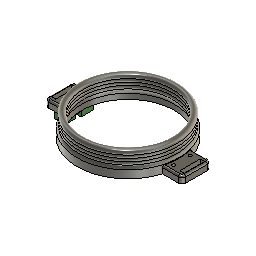
Lunette (Autodesk Fusion 360 design; units mm, degrees)
Autodesk Fusion 360 part; units mm, degrees
sketch "Sketch1" plane through (0, 0, 0) normal (0, 0, 1) x (1, 0, 0)
  circle A0 centre (0, 0) radius 64.5
  circle A1 centre (0, 0) radius 70.5
  line L0 (95, -20) -> (-95, -20)
  line L1 (-95, -20) -> (-95, 20)
  line L2 (-95, 20) -> (95, 20)
  line L3 (95, 20) -> (95, -20)
  line L4 (95, -20) -> (-95, 20) construction
  line L5 (-95, -20) -> (95, 20) construction
  line L6 (-67, 20) -> (-67, -20)
  line L7 (67, 20) -> (67, -20)
  line L8 (-83, 20) -> (-83, -20)
  line L9 (83, 20) -> (83, -20)
  line L10 (-83, 20) -> (-95, -20) construction
  line L11 (83, 20) -> (95, -20) construction
  line L12 (-86, -14) -> (-92, -14)
  line L13 (-92, -14) -> (-92, 14)
  line L14 (-92, 14) -> (-86, 14)
  line L15 (-86, 14) -> (-86, -14)
  line L16 (-86, -14) -> (-92, 14) construction
  line L17 (-92, -14) -> (-86, 14) construction
  line L18 (0, 20) -> (0, -20) construction
  line L19 (92, -14) -> (92, 14)
  line L20 (92, 14) -> (86, 14)
  line L21 (86, 14) -> (86, -14)
  line L22 (86, -14) -> (92, -14)
  line L23 (-89, 0) -> (0, 0) construction
  circle A2 centre (-75, -11.5) radius 2.1
  line L24 (-67, 20) -> (-83, -20) construction
  line L25 (-75, 20) -> (-75, -20) construction
  circle A3 centre (-75, 11.5) radius 2.1
  line L26 (75, 20) -> (75, -20) construction
  circle A4 centre (75, 11.5) radius 2.1
  circle A5 centre (75, -11.5) radius 2.1
  point P0 (-89, 0)
  dimension "d1" = 129
  dimension "d2" = 6
  dimension "d3" = 16
  dimension "d4" = 16
  dimension "d5" = 12
  dimension "d6" = 12
  dimension "d7" = 3
  dimension "d8" = 6
  dimension "d9" = 40
  dimension "d15" = 4.2
  dimension "d31" = 8.5
  dimension "d32" = 4.2
  dimension "d33" = 8.5
  dimension "d55" = 75
  dimension "d56" = 8
  constraint coincident A0.centre A1.centre
  constraint horizontal L0
  constraint perpendicular L0 L1
  constraint parallel L0 L2
  constraint parallel L1 L3
  constraint coincident L4 A0.centre
  constraint coincident L5 A0.centre
  constraint coincident L2 L6.start
  constraint coincident L0 L6.end
  constraint perpendicular L0 L6
  constraint coincident L2 L7.start
  constraint coincident L0 L7.end
  constraint perpendicular L0 L7
  constraint coincident L2 L8.start
  constraint coincident L0 L8.end
  constraint perpendicular L0 L8
  constraint coincident L2 L9.start
  constraint coincident L0 L9.end
  constraint perpendicular L0 L9
  constraint horizontal L12
  constraint perpendicular L12 L13
  constraint parallel L12 L14
  constraint parallel L13 L15
  constraint coincident L16 P0
  constraint coincident L17 P0
  constraint midpoint L10 P0
  constraint midpoint L2 L18.start
  constraint midpoint L0 L18.end
  constraint symmetric L12.start L18 L21.end
  constraint symmetric L12.end L18 L19.start
  constraint symmetric L13.end L18 L19.end
  constraint symmetric L14.end L18 L20.end
  constraint coincident P0 L23.start
  constraint coincident L2 L25.start
  constraint coincident L0 L25.end
  constraint perpendicular L0 L25
  constraint midpoint L24 L25
  constraint coincident A2.centre L25
  constraint coincident L25 A3.centre
  constraint symmetric L18 A2 A5
  constraint symmetric L18 L25.start L26.start
  constraint symmetric L18 L25.end L26.end
  constraint symmetric L18 A3 A4
  measures "d1" diameter of A0
  measures "d3" distance of L6.start L8.start
  measures "d4" distance of L7.start L9.start
  measures "d5" distance of L1 L8
  measures "d6" distance of L2.end L9.start
  measures "d7" horizontal distance of L1.end L13.end
  measures "d8" vertical distance of L1.end L13.end
  measures "d9" distance of L0.start L2.end
  measures "d15" diameter of A2
  measures "d31" distance of A2.centre L25.end
  measures "d32" diameter of A3
  measures "d33" distance of L25.start A3.centre
  measures "d55" distance of L18.start L25.start
  measures "d56" distance of L7.start L26.start
extrude "Extrude4" add sketch "Sketch1" along normal blind 15 contours A0 L0 L2 L7 | A0 A1 L2 | A0 A1 L0 | A0 L0 L2 L6 | A1 L0 L2 L7 | A1 L0 L2 L6 makes body 1
extrude "Extrude1" add sketch "Sketch1" along normal blind 10 contours A0 L0 L2 L7 | A0 A1 L2 | A0 A1 L0 | A0 L0 L2 L6 | A1 L0 L2 L7 | A1 L0 L2 L6 | A1 L0 L2 L9 | A1 L0 L2 L8 | L0 L2 L3 L9 | L0 L1 L2 L8 bodies 1
fillet "Fillet1" radius 5 4 edges at (95, -20, 5) (95, 20, 5) (-95, -20, 5) (-95, 20, 5) on bodies 1
fillet "Fillet2" radius 2.5 10 edges at (-78.8018, 20, 10) (-93.5355, 18.5355, 10) (-95, 0, 10) (-93.5355, -18.5355, 10) (-78.8018, -20, 10) (78.8018, -20, 10) (93.5355, -18.5355, 10) (95, 0, 10) (93.5355, 18.5355, 10) (78.8018, 20, 10) on bodies 1
sketch "Sketch2" plane through (0, 0, 10) normal (0, 0, 1) x (-1, 0, 0)
  line L0 (90, 17.5) -> (68.2935, 17.5)
  arc A0 (68.2935, -17.5) -> (68.2935, 17.5) centre (0, 0) ccw
  line L1 (68.2935, -17.5) -> (90, -17.5)
  arc A1 (90, -17.5) -> (92.5, -15) centre (90, -15) ccw
  line L2 (92.5, -15) -> (92.5, 15)
  arc A2 (92.5, 15) -> (90, 17.5) centre (90, 15) ccw
  circle A3 centre (75, -11.5) radius 2.1
  circle A4 centre (75, 11.5) radius 2.1
  line L3 (92, -14) -> (86, -14)
  line L4 (86, -14) -> (86, 14)
  line L5 (86, 14) -> (92, 14)
  line L6 (92, 14) -> (92, -14)
  circle A5 centre (75, 11.5) radius 3.75
  circle A6 centre (75, -11.5) radius 3.75
  line L7 (-90, -17.5) -> (-68.2935, -17.5)
  arc A7 (-68.2935, 17.5) -> (-68.2935, -17.5) centre (0, 0) ccw
  line L8 (-68.2935, 17.5) -> (-90, 17.5)
  arc A8 (-90, 17.5) -> (-92.5, 15) centre (-90, 15) ccw
  line L9 (-92.5, 15) -> (-92.5, -15)
  arc A9 (-92.5, -15) -> (-90, -17.5) centre (-90, -15) ccw
  circle A10 centre (-75, -11.5) radius 2.1
  line L10 (-92, 14) -> (-86, 14)
  line L11 (-86, 14) -> (-86, -14)
  line L12 (-86, -14) -> (-92, -14)
  line L13 (-92, -14) -> (-92, 14)
  circle A11 centre (-75, 11.5) radius 2.1
  circle A12 centre (-75, -11.5) radius 3.75
  circle A13 centre (-75, 11.5) radius 3.75
  dimension "d36" = 7.5
  dimension "d44" = 7.5
  dimension "d45" = 7.5
  dimension "d46" = 7.5
  constraint concentric A4 A5
  constraint concentric A3 A6
  constraint concentric A10 A12
  constraint concentric A11 A13
  measures "d36" diameter of A5
  measures "d44" diameter of A6
  measures "d45" diameter of A12
  measures "d46" diameter of A13
ref_plane "WorkPlane1" through (0, 0, 17) normal (0, 0, 1) x (1, 0, 0)
torus "TorusPrimitive3" add centre line diameter 130 section diameter 8 placed x (1, 0, 0) y (0, 1, 0) z (0, 0, 1) at (0, 0, 17) bodies 1
fillet "Fillet3" radius 5.5 1 edges at (-65.7291, -25.4939, 15) on bodies 1
ref_plane "WorkPlane2" through (0, 0, 21) normal (0, 0, 1) x (1, 0, 0)
torus "TorusPrimitive4" add centre line diameter 130 section diameter 8 placed x (1, 0, 0) y (0, 1, 0) z (0, 0, 1) at (0, 0, 21) bodies 1
ref_plane "WorkPlane3" through (0, 0, 25) normal (0, 0, 1) x (1, 0, 0)
torus "TorusPrimitive5" add centre line diameter 130 section diameter 8 placed x (1, 0, 0) y (0, 1, 0) z (0, 0, 1) at (0, 0, 25) bodies 1
fillet "Fillet4" radius 11 1 edges at (-60.1351, -23.3242, 13.0314) on bodies 1
ref_plane "WorkPlane4" through (0, 0, 29) normal (0, 0, 1) x (1, 0, 0)
torus "TorusPrimitive6" add centre line diameter 130 section diameter 8 placed x (1, 0, 0) y (0, 1, 0) z (0, 0, 1) at (0, 0, 29) bodies 1
sketch "Sketch16" plane through (0, 0, 0) normal (0, 0, -1) x (1, 0, 0)
  arc A0 (-95, -15) -> (-90, -20) centre (-90, -15) ccw
  line L0 (-90, -20) -> (-67.6036, -20)
  arc A1 (-67.6036, -20) -> (67.6036, -20) centre (0, 0) ccw
  line L1 (67.6036, -20) -> (90, -20)
  arc A2 (90, -20) -> (95, -15) centre (90, -15) ccw
  line L2 (95, -15) -> (95, 15)
  arc A3 (95, 15) -> (90, 20) centre (90, 15) ccw
  line L3 (90, 20) -> (67.6036, 20)
  arc A4 (67.6036, 20) -> (-67.6036, 20) centre (0, 0) ccw
  line L4 (-67.6036, 20) -> (-90, 20)
  arc A5 (-90, 20) -> (-95, 15) centre (-90, 15) ccw
  line L5 (-95, 15) -> (-95, -15)
  circle A6 centre (75, -11.5) radius 2.1
  line L6 (86, 14) -> (92, 14)
  line L7 (92, 14) -> (92, -14)
  line L8 (92, -14) -> (86, -14)
  line L9 (86, -14) -> (86, 14)
  circle A7 centre (75, 11.5) radius 2.1
  circle A8 centre (-75, -11.5) radius 2.1
  circle A9 centre (-75, 11.5) radius 2.1
  line L10 (-86, -14) -> (-92, -14)
  line L11 (-92, -14) -> (-92, 14)
  line L12 (-92, 14) -> (-86, 14)
  line L13 (-86, 14) -> (-86, -14)
  circle A10 centre (0, 0) radius 64.5
  line L14 (-75, -20) -> (-75, 20) construction
  line L15 (-82.5, 20) -> (-67.5, 20)
  line L16 (-67.5, 20) -> (-67.5, -20)
  line L17 (-67.5, -20) -> (-82.5, -20)
  line L18 (-82.5, -20) -> (-82.5, 20)
  line L19 (-82.5, 20) -> (-67.5, -20) construction
  line L20 (-67.5, 20) -> (-82.5, -20) construction
  line L21 (-82.5, -2.5) -> (-67.5, -2.5)
  line L22 (-82.5, 6) -> (-67.5, 6)
  point P0 (-75, 0)
  point P1 (-75, 0)
  dimension "d70" = 15
  dimension "d82" = 17.5
  dimension "d83" = 14
  constraint coincident L0 L14.start
  constraint coincident L4 L14.end
  constraint perpendicular L4 L14
  constraint coincident A8.centre L14
  constraint horizontal L15
  constraint perpendicular L15 L16
  constraint parallel L15 L17
  constraint parallel L16 L18
  constraint coincident L19 P1
  constraint coincident L20 P1
  constraint coincident L4 L15.start
  constraint midpoint L14 P1
  constraint coincident P1 P0
  constraint coincident L18 L21.start
  constraint coincident L16 L21.end
  constraint perpendicular L16 L21
  constraint coincident L18 L22.start
  constraint coincident L16 L22.end
  constraint perpendicular L16 L22
  measures "d70" distance of L16.end L17.end
  measures "d82" distance of L16.end L21.end
  measures "d83" distance of L15.end L22.end
extrude "Extrude9" add sketch "Sketch16" along normal blind 4 separate body contours L0 L16 L17 L18 L21 | L16 L18 L21 L22 | L4 L15 L16 L18 L22 makes body 2
extrude "Extrude11" add sketch "Sketch16" along normal blind 8.5 contours L4 L15 L16 L18 L22 bodies 2
extrude "Extrude12" add sketch "Sketch16" along normal blind 10.5 contours L0 L16 L17 L18 L21 bodies 2
named bodies: "Lunnete"
